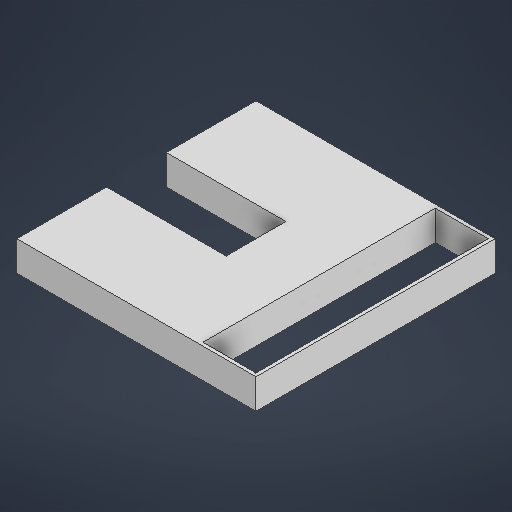
# Autodesk Inventor part: MAX30102
Saved by Autodesk Inventor 2026.1 (Build 301233000, 233)
## iProperties
Created: 2025-07-30
Part Number: MAX30102
Material: Generic
Document SubType Name: Modeling
Designer: grego
Density: 1 g/cm^3
Appearance: Default
Author: grego
Autodesk Inventor part; units mm, degrees
ref_plane "YZ Plane" through (0, 0, 0) normal (1, 0, 0) x (0, 1, 0)
ref_plane "XZ Plane" through (0, 0, 0) normal (0, 1, 0) x (-1, 0, 0)
ref_plane "XY Plane" through (0, 0, 0) normal (0, 0, 1) x (1, 0, 0)
sketch "Sketch2" plane through (0, 0, 0) normal (0, 1, 0) x (-1, 0, 0)
  line L0 (0, 0) -> (3.175, 0)
  line L1 (3.175, 0) -> (12.7, 0)
  line L2 (12.7, 0) -> (12.7, -4.7625)
  line L3 (12.7, -4.7625) -> (12.7, -7.9375)
  line L4 (12.7, -7.9375) -> (12.7, -12.7)
  line L5 (12.7, -12.7) -> (3.175, -12.7)
  line L6 (3.175, -12.7) -> (0, -12.7)
  line L7 (0, -12.7) -> (0, 0)
  line L8 (3.175, 0) -> (3.175, -12.7)
  line L9 (12.7, -4.7625) -> (6.35, -4.7625)
  line L10 (6.35, -4.7625) -> (6.35, -7.9375)
  line L11 (6.35, -7.9375) -> (12.7, -7.9375)
  line L12 (0, 0) -> (0.173, -0.173)
  line L13 (0, 0) -> (0.2447, 0) construction
  line L14 (0, -12.7) -> (0.1796, -12.5204)
  line L15 (0, -12.7) -> (0.254, -12.7) construction
  line L16 (3.175, -12.7) -> (2.9954, -12.5204)
  line L17 (3.175, 0) -> (2.9954, -0.1796)
  line L18 (3.175, 0) -> (3.429, 0) construction
  line L19 (2.9954, -0.1796) -> (2.9954, -12.5204)
  line L20 (2.9954, -12.5204) -> (0.1796, -12.5204)
  line L21 (0.1796, -12.5204) -> (0.173, -0.173)
  line L22 (2.9954, -0.1796) -> (0.173, -0.173)
  dimension "d26" = 3.175
  dimension "d27" = 9.525
  dimension "d28" = 4.7625
  dimension "d29" = 3.175
  dimension "d30" = 4.7625
  dimension "d31" = 9.525
  dimension "d32" = 3.175
  dimension "d33" = 12.7
  dimension "d34" = 6.35
  dimension "d35" = 3.175
  dimension "d36" = 45
  dimension "d37" = 0.254
  dimension "d38" = 45
  dimension "d39" = 0.254
  dimension "d40" = 0.254
  dimension "d41" = 135
  constraints: 46 end point, 5 horizontal, 4 point on line, 3 equal length, 3 perpendicular, 1 parallel, 1 vertical
  measures "d26" distance of L0.start L0.end
  measures "d27" distance of L0.end L1.end
  measures "d28" distance of L1.end L2.end
  measures "d29" distance of L2.end L3.end
  measures "d30" distance of L3.end L4.end
  measures "d31" distance of L4.end L5.end
  measures "d32" distance of L5.end L6.end
  measures "d33" distance of L6.end L0.start
  measures "d34" distance of L2.end L9.end
  measures "d35" distance of L9.end L10.end
  measures "d36" angle of L12 L13
  measures "d37" distance of L6.end L14.end
  measures "d38" angle of L15 L14
  measures "d39" distance of L5.end L16.end
  measures "d40" distance of L0.end L17.end
  measures "d41" angle of L17 L18
extrude "Extrusion1" add sketch "Sketch2" along normal blind 1.5875 contours L12 L21 L14 L7 | L0 L17 L22 L12 | L1 L2 L9 L10 L11 L4 L5 L8 | L8 L16 L19 L17 | L14 L20 L16 L6
body "Solid2"
